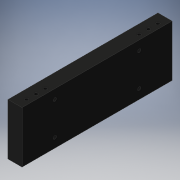
# Autodesk Inventor part: BackBatteryPlate
Saved by Autodesk Inventor 2019 (Build 230136000, 136)
## iProperties
Created: 2018-11-18
Part Number: BackBatteryPlate
Material: Generic
Document SubType Name: Modeling
Designer: james
Density: 1 g/cm^3
Appearance: Default(1)
Author: james
Autodesk Inventor part; units mm, degrees
ref_plane "YZ Plane" through (0, 0, 0) normal (1, 0, 0) x (0, 1, 0)
ref_plane "XZ Plane" through (0, 0, 0) normal (0, 1, 0) x (-1, 0, 0)
ref_plane "XY Plane" through (0, 0, 0) normal (0, 0, 1) x (1, 0, 0)
sketch "Sketch1" plane through (0, 0, 0) normal (0, 1, 0) x (-1, 0, 0)
  line L0 (17.6389, 42.7869) -> (-1.4111, 42.7869)
  line L1 (-1.4111, 42.7869) -> (-1.4111, -160.4131)
  line L2 (-1.4111, -160.4131) -> (17.6389, -160.4131)
  line L3 (17.6389, -160.4131) -> (17.6389, 42.7869)
  point P0 (0, 0)
  dimension "d0" = 19.05
  dimension "d1" = 203.2
  constraints: 8 end point, 2 parallel, 1 horizontal, 1 perpendicular
  measures "d0" distance of L0.start L0.end
  measures "d1" distance of L2.end L0.start
extrude "Extrusion1" add sketch "Sketch1" along normal blind 69.85
sketch "Sketch2" plane through (0, 69.85, 0) normal (0, 1, 0) x (1, 0, 0)
  line L0 (-17.6389, -42.7869) -> (1.4111, -42.7869) projected
  line L1 (1.4111, -42.7869) -> (1.4111, 160.4131) projected
  line L2 (1.4111, 160.4131) -> (-17.6389, 160.4131) projected
  point P0 (0, 0)
  point P1 (-4.9389, -30.0869)
  point P2 (-4.9389, -17.3869)
  point P3 (-4.9389, -4.6869)
  point P4 (-4.9389, 135.0131)
  point P5 (-4.9389, 122.3131)
  point P6 (-4.9389, 147.7131)
  dimension "d4" = 0
  dimension "d5" = 0
  dimension "d6" = 12.7
  dimension "d7" = 12.7
  dimension "d8" = 12.7
  dimension "d9" = 6.35
  dimension "d10" = 12.7
  dimension "d11" = 6.35
  dimension "d12" = 0
  dimension "d13" = 12.7
  dimension "d14" = 12.7
  dimension "d15" = 0
  measures "d4" horizontal distance of point (-4.939, -17.387) point (-4.939, -4.687)
  measures "d5" horizontal distance of point (-4.939, -30.087) point (-4.939, -17.387)
  measures "d6" distance from line of L0 point (-4.939, -30.087)
  measures "d7" distance of point (-4.939, -30.087) point (-4.939, -17.387)
  measures "d8" distance of point (-4.939, -17.387) point (-4.939, -4.687)
  measures "d9" distance from line of L1 point (-4.939, -4.687)
  measures "d10" distance from line of L2 point (-4.939, 147.713)
  measures "d11" distance from line of L1 point (-4.939, 147.713)
  measures "d12" horizontal distance of point (-4.939, 135.013) point (-4.939, 147.713)
  measures "d13" distance of point (-4.939, 135.013) point (-4.939, 147.713)
  measures "d14" distance of point (-4.939, 135.013) point (-4.939, 122.313)
  measures "d15" horizontal distance of point (-4.939, 135.013) point (-4.939, 122.313)
hole "Hole1" at (-4.9389, 69.85, 30.0869) at (-4.9389, 69.85, 17.3869) at (-4.9389, 69.85, 4.6869) at (-4.9389, 69.85, -135.0131) at (-4.9389, 69.85, -122.3131) at (-4.9389, 69.85, -147.7131) direction (0, -1, 0) diameter 4.318 end through all
sketch "Sketch3" plane through (-17.6389, 0, -160.4131) normal (-1, 0, 0) x (0, 0, 1)
  line L0 (101.6, 78.5929) -> (101.6, -10.5439)
  line L1 (0, 0) -> (0, 69.85) projected
  line L2 (203.2, 0) -> (0, 0) projected
  line L3 (0, 69.85) -> (203.2, 69.85) projected
  point P0 (160.4131, 0)
  point P1 (44.45, 57.15)
  point P2 (44.45, 12.7)
  point P3 (158.75, 57.15)
  point P4 (158.75, 12.7)
  dimension "d23" = 101.6
  dimension "d24" = 0
  dimension "d25" = 12.7
  dimension "d26" = 12.7
  dimension "d27" = 57.15
  dimension "d28" = 0
  dimension "d29" = 0
  dimension "d30" = 0
  dimension "d31" = 57.15
  constraints: 2 end point, 1 vertical
  measures "d23" distance between parallel lines of L1 L0
  measures "d24" horizontal distance of point (44.45, 12.7) point (44.45, 57.15)
  measures "d25" distance from line of L2 point (44.45, 12.7)
  measures "d26" distance from line of L3 point (44.45, 57.15)
  measures "d27" distance from line of L0 point (44.45, 57.15)
  measures "d28" horizontal distance of point (158.75, 12.7) point (158.75, 57.15)
  measures "d29" vertical distance of point (44.45, 12.7) point (158.75, 12.7)
  measures "d30" vertical distance of point (44.45, 57.15) point (158.75, 57.15)
  measures "d31" distance from line of L0 point (158.75, 57.15)
hole "Hole2" at (-17.6389, 57.15, -115.9631) at (-17.6389, 12.7, -115.9631) at (-17.6389, 57.15, -1.6631) at (-17.6389, 12.7, -1.6631) direction (1, 0, 0) diameter 4.318 depth 25.4 tip angle 118 counterbore diameter 9.525 counterbore depth 6.35
body "Solid1"
